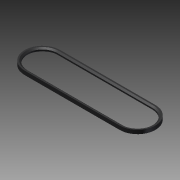
# Autodesk Inventor part: big belt
Saved by Autodesk Inventor 2011 (Build 150239000, 239)
## iProperties
Created: 2010-04-19
Part Number: big belt
Document SubType Name: Modeling
Designer: lucio
Density: 0.93 g/cm^3
Material: Rubber
Author: lucio
Autodesk Inventor part; units mm, degrees
ref_plane "YZ Plane" through (0, 0, 0) normal (1, 0, 0) x (0, 1, 0)
ref_plane "XZ Plane" through (0, 0, 0) normal (0, 1, 0) x (-1, 0, 0)
ref_plane "XY Plane" through (0, 0, 0) normal (0, 0, 1) x (1, 0, 0)
sketch "Sketch1" plane through (0, 0, 0) normal (0, 0, 1) x (1, 0, 0)
  line L0 (75, 0) -> (475, 0)
  line L1 (550, 75) -> (550, 75)
  line L2 (475, 150) -> (75, 150)
  line L3 (0, 75) -> (0, 75)
  arc A0 (75, 150) -> (0, 75) centre (75, 75) ccw
  arc A1 (0, 75) -> (75, 0) centre (75, 75) ccw
  arc A2 (475, 0) -> (550, 75) centre (475, 75) ccw
  arc A3 (550, 75) -> (475, 150) centre (475, 75) ccw
  line L4 (75, 138) -> (475, 138)
  line L5 (538, 75) -> (538, 75)
  line L6 (475, 12) -> (75, 12)
  line L7 (12, 75) -> (12, 75)
  arc A4 (75, 138) -> (12, 75) centre (75, 75) ccw
  arc A5 (12, 75) -> (75, 12) centre (75, 75) ccw
  arc A6 (475, 12) -> (538, 75) centre (475, 75) ccw
  arc A7 (538, 75) -> (475, 138) centre (475, 75) ccw
  point P0 (0, 0)
  point P1 (550, 150)
  point P2 (550, 0)
  point P3 (0, 150)
  point P4 (531, 5)
  point P5 (531, 131)
  point P6 (5, 5)
  point P7 (538, 12)
  point P8 (538, 138)
  point P9 (12, 12)
  dimension "d0" = 550
  dimension "d1" = 150
  dimension "d2" = 75
  dimension "d3" = 526
  dimension "d4" = 126
  dimension "d6" = 526
  dimension "d7" = 126
  dimension "d8" = 63
  constraints: 16 end point, 16 point on circle, 16 tangent, 14 point on line, 8 centre point, 6 equal radius, 4 parallel, 2 horizontal, 2 perpendicular, 1 coincident
  measures "d0" distance of point (0, 150) point (550, 150)
  measures "d1" distance of point (550, 150) point (550, 0)
  measures "d2" radius of A0
  measures "d3" distance of point (531, 5) point (5, 5)
  measures "d4" distance of point (531, 131) point (531, 5)
  measures "d6" distance of point (538, 12) point (12, 12)
  measures "d7" distance of point (538, 138) point (538, 12)
  measures "d8" radius of A4
extrude "Extrusion1" add sketch "Sketch1" along normal blind 16
chamfer "Chamfer1" distance 6 angle 40 6 edges at (275, 12, 16) (30.4523, 119.5477, 16) (30.4523, 30.4523, 16) (275, 138, 16) (519.5477, 30.4523, 16) (519.5477, 119.5477, 16) measured on face at (30.0987, 30.0987, 16) measured on face at (519.9013, 30.0987, 16) measured on face at (519.9013, 119.9013, 16) measured on face at (30.0987, 119.9013, 16) measured on face at (275, 11.5, 16) measured on face at (275, 138.5, 16)
chamfer "Chamfer2" distance 6 angle 40 6 edges at (275, 138, 0) (30.4523, 119.5477, 0) (30.4523, 30.4523, 0) (275, 12, 0) (519.5477, 30.4523, 0) (519.5477, 119.5477, 0) measured on face at (519.9013, 30.0987, 0) measured on face at (30.0987, 119.9013, 0) measured on face at (30.0987, 30.0987, 0) measured on face at (519.9013, 119.9013, 0) measured on face at (275, 138.5, 0) measured on face at (275, 11.5, 0)
body "Solid1"
